Autodesk Inventor part; units mm, degrees
(part 4 of 4)
  line L177 (-517.1372, 1.22) -> (-517.8628, 1.22)
  arc A519 (-517.8628, 1.22) -> (-518.1122, 0.9525) centre (-517.8628, 0.97) ccw
  arc A520 (-519.8878, 0.9525) -> (-518.1122, 0.9525) centre (-519, 0.89) ccw
  arc A521 (-519.8878, 0.9525) -> (-520.1372, 1.22) centre (-520.1372, 0.97) ccw
  line L178 (-520.1372, 1.22) -> (-520.8628, 1.22)
  arc A522 (-520.8628, 1.22) -> (-521.1122, 0.9525) centre (-520.8628, 0.97) ccw
  arc A523 (-522.8878, 0.9525) -> (-521.1122, 0.9525) centre (-522, 0.89) ccw
  arc A524 (-522.8878, 0.9525) -> (-523.1372, 1.22) centre (-523.1372, 0.97) ccw
  line L179 (-523.1372, 1.22) -> (-523.8628, 1.22)
  arc A525 (-523.8628, 1.22) -> (-524.1122, 0.9525) centre (-523.8628, 0.97) ccw
  arc A526 (-525.8878, 0.9525) -> (-524.1122, 0.9525) centre (-525, 0.89) ccw
  arc A527 (-525.8878, 0.9525) -> (-526.1372, 1.22) centre (-526.1372, 0.97) ccw
  line L180 (-526.1372, 1.22) -> (-526.8628, 1.22)
  arc A528 (-526.8628, 1.22) -> (-527.1122, 0.9525) centre (-526.8628, 0.97) ccw
  arc A529 (-528.8878, 0.9525) -> (-527.1122, 0.9525) centre (-528, 0.89) ccw
  arc A530 (-528.8878, 0.9525) -> (-529.1372, 1.22) centre (-529.1372, 0.97) ccw
  line L181 (-529.1372, 1.22) -> (-529.8628, 1.22)
  arc A531 (-529.8628, 1.22) -> (-530.1122, 0.9525) centre (-529.8628, 0.97) ccw
  arc A532 (-531.8878, 0.9525) -> (-530.1122, 0.9525) centre (-531, 0.89) ccw
  arc A533 (-531.8878, 0.9525) -> (-532.1372, 1.22) centre (-532.1372, 0.97) ccw
  line L182 (-532.1372, 1.22) -> (-532.8628, 1.22)
  arc A534 (-532.8628, 1.22) -> (-533.1122, 0.9525) centre (-532.8628, 0.97) ccw
  arc A535 (-534.8878, 0.9525) -> (-533.1122, 0.9525) centre (-534, 0.89) ccw
  arc A536 (-534.8878, 0.9525) -> (-535.1372, 1.22) centre (-535.1372, 0.97) ccw
  line L183 (-535.1372, 1.22) -> (-535.8628, 1.22)
  arc A537 (-535.8628, 1.22) -> (-536.1122, 0.9525) centre (-535.8628, 0.97) ccw
  arc A538 (-537.8878, 0.9525) -> (-536.1122, 0.9525) centre (-537, 0.89) ccw
  arc A539 (-537.8878, 0.9525) -> (-538.1372, 1.22) centre (-538.1372, 0.97) ccw
  line L184 (-538.1372, 1.22) -> (-538.8628, 1.22)
  arc A540 (-538.8628, 1.22) -> (-539.1122, 0.9525) centre (-538.8628, 0.97) ccw
  arc A541 (-540.8878, 0.9525) -> (-539.1122, 0.9525) centre (-540, 0.89) ccw
  arc A542 (-540.8878, 0.9525) -> (-541.1372, 1.22) centre (-541.1372, 0.97) ccw
  line L185 (-541.1372, 1.22) -> (-541.8628, 1.22)
  arc A543 (-541.8628, 1.22) -> (-542.1122, 0.9525) centre (-541.8628, 0.97) ccw
  arc A544 (-543.8878, 0.9525) -> (-542.1122, 0.9525) centre (-543, 0.89) ccw
  arc A545 (-543.8878, 0.9525) -> (-544.1372, 1.22) centre (-544.1372, 0.97) ccw
  line L186 (-544.1372, 1.22) -> (-544.8628, 1.22)
  arc A546 (-544.8628, 1.22) -> (-545.1122, 0.9525) centre (-544.8628, 0.97) ccw
  arc A547 (-546.8878, 0.9525) -> (-545.1122, 0.9525) centre (-546, 0.89) ccw
  arc A548 (-546.8878, 0.9525) -> (-547.1372, 1.22) centre (-547.1372, 0.97) ccw
  line L187 (-547.1372, 1.22) -> (-547.8628, 1.22)
  arc A549 (-547.8628, 1.22) -> (-548.1122, 0.9525) centre (-547.8628, 0.97) ccw
  arc A550 (-549.8878, 0.9525) -> (-548.1122, 0.9525) centre (-549, 0.89) ccw
  arc A551 (-549.8878, 0.9525) -> (-550.1372, 1.22) centre (-550.1372, 0.97) ccw
  line L188 (-550.1372, 1.22) -> (-550.8628, 1.22)
  arc A552 (-550.8628, 1.22) -> (-551.1122, 0.9525) centre (-550.8628, 0.97) ccw
  arc A553 (-552.8878, 0.9525) -> (-551.1122, 0.9525) centre (-552, 0.89) ccw
  arc A554 (-552.8878, 0.9525) -> (-553.1372, 1.22) centre (-553.1372, 0.97) ccw
  line L189 (-553.1372, 1.22) -> (-553.8628, 1.22)
  arc A555 (-553.8628, 1.22) -> (-554.1122, 0.9525) centre (-553.8628, 0.97) ccw
  arc A556 (-555.8878, 0.9525) -> (-554.1122, 0.9525) centre (-555, 0.89) ccw
  arc A557 (-555.8878, 0.9525) -> (-556.1372, 1.22) centre (-556.1372, 0.97) ccw
  line L190 (-556.1372, 1.22) -> (-556.8628, 1.22)
  arc A558 (-556.8628, 1.22) -> (-557.1122, 0.9525) centre (-556.8628, 0.97) ccw
  arc A559 (-558.8878, 0.9525) -> (-557.1122, 0.9525) centre (-558, 0.89) ccw
  arc A560 (-558.8878, 0.9525) -> (-559.1372, 1.22) centre (-559.1372, 0.97) ccw
  line L191 (-559.1372, 1.22) -> (-559.8628, 1.22)
  arc A561 (-559.8628, 1.22) -> (-560.1122, 0.9525) centre (-559.8628, 0.97) ccw
  arc A562 (-561.8878, 0.9525) -> (-560.1122, 0.9525) centre (-561, 0.89) ccw
  arc A563 (-561.8878, 0.9525) -> (-562.1372, 1.22) centre (-562.1372, 0.97) ccw
  line L192 (-562.1372, 1.22) -> (-562.8628, 1.22)
  arc A564 (-562.8628, 1.22) -> (-563.1122, 0.9525) centre (-562.8628, 0.97) ccw
  arc A565 (-564.8878, 0.9525) -> (-563.1122, 0.9525) centre (-564, 0.89) ccw
  arc A566 (-564.8878, 0.9525) -> (-565.1372, 1.22) centre (-565.1372, 0.97) ccw
  line L193 (-565.1372, 1.22) -> (-565.8628, 1.22)
  arc A567 (-565.8628, 1.22) -> (-566.1122, 0.9525) centre (-565.8628, 0.97) ccw
  arc A568 (-567.8878, 0.9525) -> (-566.1122, 0.9525) centre (-567, 0.89) ccw
  arc A569 (-567.8878, 0.9525) -> (-568.1372, 1.22) centre (-568.1372, 0.97) ccw
  line L194 (-568.1372, 1.22) -> (-568.8628, 1.22)
  arc A570 (-568.8628, 1.22) -> (-569.1122, 0.9525) centre (-568.8628, 0.97) ccw
  arc A571 (-570.8878, 0.9525) -> (-569.1122, 0.9525) centre (-570, 0.89) ccw
  arc A572 (-570.8878, 0.9525) -> (-571.1372, 1.22) centre (-571.1372, 0.97) ccw
  line L195 (-571.1372, 1.22) -> (-571.8628, 1.22)
  arc A573 (-571.8628, 1.22) -> (-572.1122, 0.9525) centre (-571.8628, 0.97) ccw
  arc A574 (-573.8878, 0.9525) -> (-572.1122, 0.9525) centre (-573, 0.89) ccw
  arc A575 (-573.8878, 0.9525) -> (-574.1372, 1.22) centre (-574.1372, 0.97) ccw
  line L196 (-574.1372, 1.22) -> (-574.8628, 1.22)
  arc A576 (-574.8628, 1.22) -> (-575.1122, 0.9525) centre (-574.8628, 0.97) ccw
  arc A577 (-576.8878, 0.9525) -> (-575.1122, 0.9525) centre (-576, 0.89) ccw
  arc A578 (-576.8878, 0.9525) -> (-577.1372, 1.22) centre (-577.1372, 0.97) ccw
  line L197 (-577.1372, 1.22) -> (-577.8628, 1.22)
  arc A579 (-577.8628, 1.22) -> (-578.1122, 0.9525) centre (-577.8628, 0.97) ccw
  arc A580 (-579.8878, 0.9525) -> (-578.1122, 0.9525) centre (-579, 0.89) ccw
  arc A581 (-579.8878, 0.9525) -> (-580.1372, 1.22) centre (-580.1372, 0.97) ccw
  line L198 (-580.1372, 1.22) -> (-580.8628, 1.22)
  arc A582 (-580.8628, 1.22) -> (-581.1122, 0.9525) centre (-580.8628, 0.97) ccw
  arc A583 (-582.8878, 0.9525) -> (-581.1122, 0.9525) centre (-582, 0.89) ccw
  arc A584 (-582.8878, 0.9525) -> (-583.1372, 1.22) centre (-583.1372, 0.97) ccw
  line L199 (-583.1372, 1.22) -> (-583.8628, 1.22)
  arc A585 (-583.8628, 1.22) -> (-584.1122, 0.9525) centre (-583.8628, 0.97) ccw
  arc A586 (-585.8878, 0.9525) -> (-584.1122, 0.9525) centre (-585, 0.89) ccw
  arc A587 (-585.8878, 0.9525) -> (-586.1372, 1.22) centre (-586.1372, 0.97) ccw
  line L200 (-586.1372, 1.22) -> (-586.8628, 1.22)
  arc A588 (-586.8628, 1.22) -> (-587.1122, 0.9525) centre (-586.8628, 0.97) ccw
  arc A589 (-588.8878, 0.9525) -> (-587.1122, 0.9525) centre (-588, 0.89) ccw
  arc A590 (-588.8878, 0.9525) -> (-589.1372, 1.22) centre (-589.1372, 0.97) ccw
  line L201 (-589.1372, 1.22) -> (-589.8628, 1.22)
  arc A591 (-589.8628, 1.22) -> (-590.1122, 0.9525) centre (-589.8628, 0.97) ccw
  arc A592 (-591.8878, 0.9525) -> (-590.1122, 0.9525) centre (-591, 0.89) ccw
  arc A593 (-591.8878, 0.9525) -> (-592.1372, 1.22) centre (-592.1372, 0.97) ccw
  line L202 (-592.1372, 1.22) -> (-592.8628, 1.22)
  arc A594 (-592.8628, 1.22) -> (-593.1122, 0.9525) centre (-592.8628, 0.97) ccw
  arc A595 (-594.8878, 0.9525) -> (-593.1122, 0.9525) centre (-594, 0.89) ccw
  arc A596 (-594.8878, 0.9525) -> (-595.1372, 1.22) centre (-595.1372, 0.97) ccw
  line L203 (-595.1372, 1.22) -> (-595.8628, 1.22)
  arc A597 (-595.8628, 1.22) -> (-596.1122, 0.9525) centre (-595.8628, 0.97) ccw
  arc A598 (-597.8878, 0.9525) -> (-596.1122, 0.9525) centre (-597, 0.89) ccw
  arc A599 (-597.8878, 0.9525) -> (-598.1372, 1.22) centre (-598.1372, 0.97) ccw
  line L204 (-598.1372, 1.22) -> (-598.8628, 1.22)
  arc A600 (-598.8628, 1.22) -> (-599.1122, 0.9525) centre (-598.8628, 0.97) ccw
  arc A601 (-600.8878, 0.9525) -> (-599.1122, 0.9525) centre (-600, 0.89) ccw
  arc A602 (-600.8878, 0.9525) -> (-601.1372, 1.22) centre (-601.1372, 0.97) ccw
  line L205 (-601.1372, 1.22) -> (-601.8628, 1.22)
  arc A603 (-601.8628, 1.22) -> (-602.1122, 0.9525) centre (-601.8628, 0.97) ccw
  arc A604 (-603.8878, 0.9525) -> (-602.1122, 0.9525) centre (-603, 0.89) ccw
  arc A605 (-603.8878, 0.9525) -> (-604.1372, 1.22) centre (-604.1372, 0.97) ccw
  line L206 (-604.1372, 1.22) -> (-604.8628, 1.22)
  arc A606 (-604.8628, 1.22) -> (-605.1122, 0.9525) centre (-604.8628, 0.97) ccw
  arc A607 (-606.8878, 0.9525) -> (-605.1122, 0.9525) centre (-606, 0.89) ccw
  arc A608 (-606.8878, 0.9525) -> (-607.1372, 1.22) centre (-607.1372, 0.97) ccw
  line L207 (-607.1372, 1.22) -> (-607.8628, 1.22)
  arc A609 (-607.8628, 1.22) -> (-608.1122, 0.9525) centre (-607.8628, 0.97) ccw
  arc A610 (-609.8878, 0.9525) -> (-608.1122, 0.9525) centre (-609, 0.89) ccw
  arc A611 (-609.8878, 0.9525) -> (-610.1372, 1.22) centre (-610.1372, 0.97) ccw
  line L208 (-610.1372, 1.22) -> (-610.8628, 1.22)
  arc A612 (-610.8628, 1.22) -> (-611.1122, 0.9525) centre (-610.8628, 0.97) ccw
  arc A613 (-612.8878, 0.9525) -> (-611.1122, 0.9525) centre (-612, 0.89) ccw
  arc A614 (-612.8878, 0.9525) -> (-613.1372, 1.22) centre (-613.1372, 0.97) ccw
  line L209 (-613.1372, 1.22) -> (-613.8628, 1.22)
  arc A615 (-613.8628, 1.22) -> (-614.1122, 0.9525) centre (-613.8628, 0.97) ccw
  arc A616 (-615.8878, 0.9525) -> (-614.1122, 0.9525) centre (-615, 0.89) ccw
  arc A617 (-615.8878, 0.9525) -> (-616.1372, 1.22) centre (-616.1372, 0.97) ccw
  line L210 (-616.1372, 1.22) -> (-616.8628, 1.22)
  arc A618 (-616.8628, 1.22) -> (-617.1122, 0.9525) centre (-616.8628, 0.97) ccw
  arc A619 (-618.8878, 0.9525) -> (-617.1122, 0.9525) centre (-618, 0.89) ccw
  arc A620 (-618.8878, 0.9525) -> (-619.1372, 1.22) centre (-619.1372, 0.97) ccw
  line L211 (-619.1372, 1.22) -> (-619.8628, 1.22)
  arc A621 (-619.8628, 1.22) -> (-620.1122, 0.9525) centre (-619.8628, 0.97) ccw
  arc A622 (-621.8878, 0.9525) -> (-620.1122, 0.9525) centre (-621, 0.89) ccw
  arc A623 (-621.8878, 0.9525) -> (-622.1372, 1.22) centre (-622.1372, 0.97) ccw
  line L212 (-622.1372, 1.22) -> (-622.8628, 1.22)
  arc A624 (-622.8628, 1.22) -> (-623.1122, 0.9525) centre (-622.8628, 0.97) ccw
  arc A625 (-624.8878, 0.9525) -> (-623.1122, 0.9525) centre (-624, 0.89) ccw
  arc A626 (-624.8878, 0.9525) -> (-625.1372, 1.22) centre (-625.1372, 0.97) ccw
  line L213 (-625.1372, 1.22) -> (-625.8628, 1.22)
  arc A627 (-625.8628, 1.22) -> (-626.1122, 0.9525) centre (-625.8628, 0.97) ccw
  arc A628 (-627.8878, 0.9525) -> (-626.1122, 0.9525) centre (-627, 0.89) ccw
  arc A629 (-627.8878, 0.9525) -> (-628.1372, 1.22) centre (-628.1372, 0.97) ccw
  line L214 (-628.1372, 1.22) -> (-628.8628, 1.22)
  arc A630 (-628.8628, 1.22) -> (-629.1122, 0.9525) centre (-628.8628, 0.97) ccw
  arc A631 (-630.8878, 0.9525) -> (-629.1122, 0.9525) centre (-630, 0.89) ccw
  arc A632 (-630.8878, 0.9525) -> (-631.1372, 1.22) centre (-631.1372, 0.97) ccw
  line L215 (-631.1372, 1.22) -> (-631.8628, 1.22)
  arc A633 (-631.8628, 1.22) -> (-632.1122, 0.9525) centre (-631.8628, 0.97) ccw
  arc A634 (-633.8878, 0.9525) -> (-632.1122, 0.9525) centre (-633, 0.89) ccw
  arc A635 (-633.8878, 0.9525) -> (-634.1372, 1.22) centre (-634.1372, 0.97) ccw
  line L216 (-634.1372, 1.22) -> (-634.8628, 1.22)
  arc A636 (-634.8628, 1.22) -> (-635.1122, 0.9525) centre (-634.8628, 0.97) ccw
  arc A637 (-636.8878, 0.9525) -> (-635.1122, 0.9525) centre (-636, 0.89) ccw
  arc A638 (-636.8878, 0.9525) -> (-637.1372, 1.22) centre (-637.1372, 0.97) ccw
  line L217 (-637.1372, 1.22) -> (-637.8628, 1.22)
  arc A639 (-637.8628, 1.22) -> (-638.1122, 0.9525) centre (-637.8628, 0.97) ccw
  arc A640 (-639.8878, 0.9525) -> (-638.1122, 0.9525) centre (-639, 0.89) ccw
  arc A641 (-639.8878, 0.9525) -> (-640.1372, 1.22) centre (-640.1372, 0.97) ccw
  line L218 (-640.1372, 1.22) -> (-640.8628, 1.22)
  arc A642 (-640.8628, 1.22) -> (-641.1122, 0.9525) centre (-640.8628, 0.97) ccw
  arc A643 (-642.8878, 0.9525) -> (-641.1122, 0.9525) centre (-642, 0.89) ccw
  arc A644 (-642.8878, 0.9525) -> (-643.1372, 1.22) centre (-643.1372, 0.97) ccw
  line L219 (-643.1372, 1.22) -> (-643.8628, 1.22)
  arc A645 (-643.8628, 1.22) -> (-644.1122, 0.9525) centre (-643.8628, 0.97) ccw
  arc A646 (-645.8878, 0.9525) -> (-644.1122, 0.9525) centre (-645, 0.89) ccw
  arc A647 (-645.8878, 0.9525) -> (-646.1372, 1.22) centre (-646.1372, 0.97) ccw
  line L220 (-646.1372, 1.22) -> (-646.8628, 1.22)
  arc A648 (-646.8628, 1.22) -> (-647.1122, 0.9525) centre (-646.8628, 0.97) ccw
  arc A649 (-648.8878, 0.9525) -> (-647.1122, 0.9525) centre (-648, 0.89) ccw
  arc A650 (-648.8878, 0.9525) -> (-649.1372, 1.22) centre (-649.1372, 0.97) ccw
  line L221 (-649.1372, 1.22) -> (-649.8628, 1.22)
  arc A651 (-649.8628, 1.22) -> (-650.1122, 0.9525) centre (-649.8628, 0.97) ccw
  arc A652 (-651.8878, 0.9525) -> (-650.1122, 0.9525) centre (-651, 0.89) ccw
  arc A653 (-651.8878, 0.9525) -> (-652.1372, 1.22) centre (-652.1372, 0.97) ccw
  line L222 (-652.1372, 1.22) -> (-652.8628, 1.22)
  arc A654 (-652.8628, 1.22) -> (-653.1122, 0.9525) centre (-652.8628, 0.97) ccw
  arc A655 (-654.8878, 0.9525) -> (-653.1122, 0.9525) centre (-654, 0.89) ccw
  arc A656 (-654.8878, 0.9525) -> (-655.1372, 1.22) centre (-655.1372, 0.97) ccw
  line L223 (-655.1372, 1.22) -> (-655.8628, 1.22)
  arc A657 (-655.8628, 1.22) -> (-656.1122, 0.9525) centre (-655.8628, 0.97) ccw
  arc A658 (-657.8878, 0.9525) -> (-656.1122, 0.9525) centre (-657, 0.89) ccw
  arc A659 (-657.8878, 0.9525) -> (-658.1372, 1.22) centre (-658.1372, 0.97) ccw
  line L224 (-658.1372, 1.22) -> (-658.8628, 1.22)
  arc A660 (-658.8628, 1.22) -> (-659.1122, 0.9525) centre (-658.8628, 0.97) ccw
  arc A661 (-660.8878, 0.9525) -> (-659.1122, 0.9525) centre (-660, 0.89) ccw
  arc A662 (-660.8878, 0.9525) -> (-661.1372, 1.22) centre (-661.1372, 0.97) ccw
  line L225 (-661.1372, 1.22) -> (-661.8628, 1.22)
  arc A663 (-661.8628, 1.22) -> (-662.1122, 0.9525) centre (-661.8628, 0.97) ccw
  arc A664 (-663.8878, 0.9525) -> (-662.1122, 0.9525) centre (-663, 0.89) ccw
  arc A665 (-663.8878, 0.9525) -> (-664.1372, 1.22) centre (-664.1372, 0.97) ccw
  line L226 (-664.1372, 1.22) -> (-664.8628, 1.22)
  arc A666 (-664.8628, 1.22) -> (-665.1122, 0.9525) centre (-664.8628, 0.97) ccw
  arc A667 (-666.8878, 0.9525) -> (-665.1122, 0.9525) centre (-666, 0.89) ccw
  arc A668 (-666.8878, 0.9525) -> (-667.1372, 1.22) centre (-667.1372, 0.97) ccw
  line L227 (-667.1372, 1.22) -> (-667.8628, 1.22)
  arc A669 (-667.8628, 1.22) -> (-668.1122, 0.9525) centre (-667.8628, 0.97) ccw
  arc A670 (-669.8878, 0.9525) -> (-668.1122, 0.9525) centre (-669, 0.89) ccw
  arc A671 (-669.8878, 0.9525) -> (-670.1372, 1.22) centre (-670.1372, 0.97) ccw
  line L228 (-670.1372, 1.22) -> (-670.8628, 1.22)
  arc A672 (-670.8628, 1.22) -> (-671.1122, 0.9525) centre (-670.8628, 0.97) ccw
  arc A673 (-672.8878, 0.9525) -> (-671.1122, 0.9525) centre (-672, 0.89) ccw
  arc A674 (-672.8878, 0.9525) -> (-673.1372, 1.22) centre (-673.1372, 0.97) ccw
  line L229 (-673.1372, 1.22) -> (-673.8628, 1.22)
  arc A675 (-673.8628, 1.22) -> (-674.1122, 0.9525) centre (-673.8628, 0.97) ccw
  arc A676 (-675.8878, 0.9525) -> (-674.1122, 0.9525) centre (-675, 0.89) ccw
  arc A677 (-675.8878, 0.9525) -> (-676.1372, 1.22) centre (-676.1372, 0.97) ccw
  line L230 (-676.1372, 1.22) -> (-676.8628, 1.22)
  arc A678 (-676.8628, 1.22) -> (-677.1122, 0.9525) centre (-676.8628, 0.97) ccw
  arc A679 (-678.8878, 0.9525) -> (-677.1122, 0.9525) centre (-678, 0.89) ccw
  arc A680 (-678.8878, 0.9525) -> (-679.1372, 1.22) centre (-679.1372, 0.97) ccw
  line L231 (-679.1372, 1.22) -> (-679.8628, 1.22)
  arc A681 (-679.8628, 1.22) -> (-680.1122, 0.9525) centre (-679.8628, 0.97) ccw
  arc A682 (-681.8878, 0.9525) -> (-680.1122, 0.9525) centre (-681, 0.89) ccw
  arc A683 (-681.8878, 0.9525) -> (-682.1372, 1.22) centre (-682.1372, 0.97) ccw
  line L232 (-682.1372, 1.22) -> (-682.8628, 1.22)
  arc A684 (-682.8628, 1.22) -> (-683.1122, 0.9525) centre (-682.8628, 0.97) ccw
  arc A685 (-684.8878, 0.9525) -> (-683.1122, 0.9525) centre (-684, 0.89) ccw
  arc A686 (-684.8878, 0.9525) -> (-685.1372, 1.22) centre (-685.1372, 0.97) ccw
  line L233 (-685.1372, 1.22) -> (-685.8628, 1.22)
  arc A687 (-685.8628, 1.22) -> (-686.1122, 0.9525) centre (-685.8628, 0.97) ccw
  arc A688 (-687.8878, 0.9525) -> (-686.1122, 0.9525) centre (-687, 0.89) ccw
  arc A689 (-687.8878, 0.9525) -> (-688.1372, 1.22) centre (-688.1372, 0.97) ccw
  line L234 (-688.1372, 1.22) -> (-688.8628, 1.22)
  arc A690 (-688.8628, 1.22) -> (-689.1122, 0.9525) centre (-688.8628, 0.97) ccw
  arc A691 (-690.8878, 0.9525) -> (-689.1122, 0.9525) centre (-690, 0.89) ccw
  arc A692 (-690.8878, 0.9525) -> (-691.1372, 1.22) centre (-691.1372, 0.97) ccw
  line L235 (-691.1372, 1.22) -> (-691.8628, 1.22)
  arc A693 (-691.8628, 1.22) -> (-692.1122, 0.9525) centre (-691.8628, 0.97) ccw
  arc A694 (-693.8878, 0.9525) -> (-692.1122, 0.9525) centre (-693, 0.89) ccw
  arc A695 (-693.8878, 0.9525) -> (-694.1372, 1.22) centre (-694.1372, 0.97) ccw
  line L236 (-694.1372, 1.22) -> (-694.8628, 1.22)
  arc A696 (-694.8628, 1.22) -> (-695.1122, 0.9525) centre (-694.8628, 0.97) ccw
  arc A697 (-696.8878, 0.9525) -> (-695.1122, 0.9525) centre (-696, 0.89) ccw
  arc A698 (-696.8878, 0.9525) -> (-697.1372, 1.22) centre (-697.1372, 0.97) ccw
  line L237 (-697.1372, 1.22) -> (-697.8628, 1.22)
  arc A699 (-697.8628, 1.22) -> (-698.1122, 0.9525) centre (-697.8628, 0.97) ccw
  arc A700 (-699.8878, 0.9525) -> (-698.1122, 0.9525) centre (-699, 0.89) ccw
  arc A701 (-699.8878, 0.9525) -> (-700.1372, 1.22) centre (-700.1372, 0.97) ccw
  line L238 (-700.1372, 1.22) -> (-700.8628, 1.22)
  arc A702 (-700.8628, 1.22) -> (-701.1122, 0.9525) centre (-700.8628, 0.97) ccw
  arc A703 (-702.8878, 0.9525) -> (-701.1122, 0.9525) centre (-702, 0.89) ccw
  arc A704 (-702.8878, 0.9525) -> (-703.1372, 1.22) centre (-703.1372, 0.97) ccw
  line L239 (-703.1372, 1.22) -> (-703.8628, 1.22)
  arc A705 (-703.8628, 1.22) -> (-704.1122, 0.9525) centre (-703.8628, 0.97) ccw
  arc A706 (-705.8878, 0.9525) -> (-704.1122, 0.9525) centre (-705, 0.89) ccw
  arc A707 (-705.8878, 0.9525) -> (-706.1372, 1.22) centre (-706.1372, 0.97) ccw
  line L240 (-706.1372, 1.22) -> (-706.8628, 1.22)
  arc A708 (-706.8628, 1.22) -> (-707.1122, 0.9525) centre (-706.8628, 0.97) ccw
  arc A709 (-708.8878, 0.9525) -> (-707.1122, 0.9525) centre (-708, 0.89) ccw
  arc A710 (-708.8878, 0.9525) -> (-709.1372, 1.22) centre (-709.1372, 0.97) ccw
  line L241 (-709.1372, 1.22) -> (-709.8628, 1.22)
  arc A711 (-709.8628, 1.22) -> (-710.1122, 0.9525) centre (-709.8628, 0.97) ccw
  arc A712 (-711.8878, 0.9525) -> (-710.1122, 0.9525) centre (-711, 0.89) ccw
  arc A713 (-711.8878, 0.9525) -> (-712.1372, 1.22) centre (-712.1372, 0.97) ccw
  line L242 (-712.1372, 1.22) -> (-712.8628, 1.22)
  arc A714 (-712.8628, 1.22) -> (-713.1122, 0.9525) centre (-712.8628, 0.97) ccw
  arc A715 (-714.8878, 0.9525) -> (-713.1122, 0.9525) centre (-714, 0.89) ccw
  arc A716 (-714.8878, 0.9525) -> (-715.1372, 1.22) centre (-715.1372, 0.97) ccw
  line L243 (-715.1372, 1.22) -> (-715.8628, 1.22)
  arc A717 (-715.8628, 1.22) -> (-716.1122, 0.9525) centre (-715.8628, 0.97) ccw
  arc A718 (-717.8878, 0.9525) -> (-716.1122, 0.9525) centre (-717, 0.89) ccw
  arc A719 (-717.8878, 0.9525) -> (-718.1372, 1.22) centre (-718.1372, 0.97) ccw
  line L244 (-718.1372, 1.22) -> (-718.8628, 1.22)
  arc A720 (-718.8628, 1.22) -> (-719.1122, 0.9525) centre (-718.8628, 0.97) ccw
  arc A721 (-720.8878, 0.9525) -> (-719.1122, 0.9525) centre (-720, 0.89) ccw
  arc A722 (-720.8878, 0.9525) -> (-721.1372, 1.22) centre (-721.1372, 0.97) ccw
  line L245 (-721.1372, 1.22) -> (-721.8628, 1.22)
  arc A723 (-721.8628, 1.22) -> (-722.1122, 0.9525) centre (-721.8628, 0.97) ccw
  arc A724 (-723.8878, 0.9525) -> (-722.1122, 0.9525) centre (-723, 0.89) ccw
  arc A725 (-723.8878, 0.9525) -> (-724.1372, 1.22) centre (-724.1372, 0.97) ccw
  line L246 (-724.1372, 1.22) -> (-724.8628, 1.22)
  arc A726 (-724.8628, 1.22) -> (-725.1122, 0.9525) centre (-724.8628, 0.97) ccw
  arc A727 (-726.8878, 0.9525) -> (-725.1122, 0.9525) centre (-726, 0.89) ccw
  arc A728 (-726.8878, 0.9525) -> (-727.1372, 1.22) centre (-727.1372, 0.97) ccw
  line L247 (-727.1372, 1.22) -> (-727.8628, 1.22)
  arc A729 (-727.8628, 1.22) -> (-728.1122, 0.9525) centre (-727.8628, 0.97) ccw
  arc A730 (-729.8878, 0.9525) -> (-728.1122, 0.9525) centre (-729, 0.89) ccw
  arc A731 (-729.8878, 0.9525) -> (-730.1372, 1.22) centre (-730.1372, 0.97) ccw
  line L248 (-730.1372, 1.22) -> (-730.8628, 1.22)
  arc A732 (-730.8628, 1.22) -> (-731.1122, 0.9525) centre (-730.8628, 0.97) ccw
  arc A733 (-732.8878, 0.9525) -> (-731.1122, 0.9525) centre (-732, 0.89) ccw
  arc A734 (-732.8878, 0.9525) -> (-733.1372, 1.22) centre (-733.1372, 0.97) ccw
  line L249 (-733.1372, 1.22) -> (-733.8628, 1.22)
  arc A735 (-733.8628, 1.22) -> (-734.1122, 0.9525) centre (-733.8628, 0.97) ccw
  arc A736 (-735.8878, 0.9525) -> (-734.1122, 0.9525) centre (-735, 0.89) ccw
  arc A737 (-735.8878, 0.9525) -> (-736.1372, 1.22) centre (-736.1372, 0.97) ccw
  line L250 (-736.1372, 1.22) -> (-736.8628, 1.22)
  arc A738 (-736.8628, 1.22) -> (-737.1122, 0.9525) centre (-736.8628, 0.97) ccw
  arc A739 (-738.8878, 0.9525) -> (-737.1122, 0.9525) centre (-738, 0.89) ccw
  arc A740 (-738.8878, 0.9525) -> (-739.1372, 1.22) centre (-739.1372, 0.97) ccw
  line L251 (-739.1372, 1.22) -> (-739.8628, 1.22)
  arc A741 (-739.8628, 1.22) -> (-740.1122, 0.9525) centre (-739.8628, 0.97) ccw
  arc A742 (-741.8878, 0.9525) -> (-740.1122, 0.9525) centre (-741, 0.89) ccw
  arc A743 (-741.8878, 0.9525) -> (-742.1372, 1.22) centre (-742.1372, 0.97) ccw
  line L252 (-742.1372, 1.22) -> (-742.8628, 1.22)
  arc A744 (-742.8628, 1.22) -> (-743.1122, 0.9525) centre (-742.8628, 0.97) ccw
  arc A745 (-744.8878, 0.9525) -> (-743.1122, 0.9525) centre (-744, 0.89) ccw
  arc A746 (-744.8878, 0.9525) -> (-745.1372, 1.22) centre (-745.1372, 0.97) ccw
  line L253 (-745.1372, 1.22) -> (-745.8628, 1.22)
  arc A747 (-745.8628, 1.22) -> (-746.1122, 0.9525) centre (-745.8628, 0.97) ccw
  arc A748 (-747.8878, 0.9525) -> (-746.1122, 0.9525) centre (-747, 0.89) ccw
  arc A749 (-747.8878, 0.9525) -> (-748.1372, 1.22) centre (-748.1372, 0.97) ccw
  line L254 (-748.1372, 1.22) -> (-748.8628, 1.22)
  arc A750 (-748.8628, 1.22) -> (-749.1122, 0.9525) centre (-748.8628, 0.97) ccw
  arc A751 (-750.8878, 0.9525) -> (-749.1122, 0.9525) centre (-750, 0.89) ccw
  arc A752 (-750.8878, 0.9525) -> (-751.1372, 1.22) centre (-751.1372, 0.97) ccw
  line L255 (-751.1372, 1.22) -> (-751.8628, 1.22)
  arc A753 (-751.8628, 1.22) -> (-752.1122, 0.9525) centre (-751.8628, 0.97) ccw
  arc A754 (-753.8878, 0.9525) -> (-752.1122, 0.9525) centre (-753, 0.89) ccw
  arc A755 (-753.8878, 0.9525) -> (-754.1372, 1.22) centre (-754.1372, 0.97) ccw
  line L256 (-754.1372, 1.22) -> (-754.8628, 1.22)
  arc A756 (-754.8628, 1.22) -> (-755.1122, 0.9525) centre (-754.8628, 0.97) ccw
  arc A757 (-756.8878, 0.9525) -> (-755.1122, 0.9525) centre (-756, 0.89) ccw
  arc A758 (-756.8878, 0.9525) -> (-757.1372, 1.22) centre (-757.1372, 0.97) ccw
  line L257 (-757.1372, 1.22) -> (-757.8628, 1.22)
  arc A759 (-757.8628, 1.22) -> (-758.1122, 0.9525) centre (-757.8628, 0.97) ccw
  arc A760 (-759.8878, 0.9525) -> (-758.1122, 0.9525) centre (-759, 0.89) ccw
  arc A761 (-759.8878, 0.9525) -> (-760.1372, 1.22) centre (-760.1372, 0.97) ccw
  line L258 (-760.1372, 1.22) -> (-760.8628, 1.22)
  arc A762 (-760.8628, 1.22) -> (-761.1122, 0.9525) centre (-760.8628, 0.97) ccw
  arc A763 (-762.8878, 0.9525) -> (-761.1122, 0.9525) centre (-762, 0.89) ccw
  arc A764 (-762.8878, 0.9525) -> (-763.1372, 1.22) centre (-763.1372, 0.97) ccw
  line L259 (-763.1372, 1.22) -> (-763.8628, 1.22)
  arc A765 (-763.8628, 1.22) -> (-764.1122, 0.9525) centre (-763.8628, 0.97) ccw
  arc A766 (-765.8878, 0.9525) -> (-764.1122, 0.9525) centre (-765, 0.89) ccw
  arc A767 (-765.8878, 0.9525) -> (-766.1372, 1.22) centre (-766.1372, 0.97) ccw
  line L260 (-766.1372, 1.22) -> (-766.8628, 1.22)
  arc A768 (-766.8628, 1.22) -> (-767.1122, 0.9525) centre (-766.8628, 0.97) ccw
  arc A769 (-768, 0) -> (-767.1122, 0.9525) centre (-768, 0.89) ccw
  point P0 (0, 0)
  constraints: 899 symmetric about line, 770 point on circle, 385 centre point, 260 end point, 385 other
extrude "Extrusion3" add sketch "Sketch3" against normal blind 15 contours L2 A385 A386 L133 A387 A388 A389 L134 A390 A391 A392 L135 A393 A394 A395 L136 A396 A397 A398 L137 A399 A400 A401 L138 A402 A403 A404 L139 A405 A406 A407 L140 A408 A409 A410 L141 A411 A412 A413 L142 A414 A415 A416 L143 A417 A418 A419 L144 A420 A421 A422 L145 A423 A424 A425 L146 A426 A427 A428 L147 A429 A430 A431 L148 A432 A433 A434 L149 A435 A436 A437 L150 A438 A439 A440 L151 A441 A442 A443 L152 A444 A445 A446 L153 A447 A448 A449 L154 A450 A451 A452 L155 A453 A454 A455 L156 A456 A457 A458 L157 A459 A460 A461 L158 A462 A463 A464 L159 A465 A466 A467 L160 A468 A469 A470 L161 A471 A472 A473 L162 A474 A475 A476 L163 A477 A478 A479 L164 A480 A481 A482 L165 A483 A484 A485 L166 A486 A487 A488 L167 A489 A490 A491 L168 A492 A493 A494 L169 A495 A496 A497 L170 A498 A499 A500 L171 A501 A502 A503 L172 A504 A505 A506 L173 A507 A508 A509 L174 A510 A511 A512 L175 A513 A514 A515 L176 A516 A517 A518 L177 A519 A520 A521 L178 A522 A523 A524 L179 A525 A526 A527 L180 A528 A529 A530 L181 A531 A532 A533 L182 A534 A535 A536 L183 A537 A538 A539 L184 A540 A541 A542 L185 A543 A544 A545 L186 A546 A547 A548 L187 A549 A550 A551 L188 A552 A553 A554 L189 A555 A556 A557 L190 A558 A559 A560 L191 A561 A562 A563 L192 A564 A565 A566 L193 A567 A568 A569 L194 A570 A571 A572 L195 A573 A574 A575 L196 A576 A577 A578 L197 A579 A580 A581 L198 A582 A583 A584 L199 A585 A586 A587 L200 A588 A589 A590 L201 A591 A592 A593 L202 A594 A595 A596 L203 A597 A598 A599 L204 A600 A601 A602 L205 A603 A604 A605 L206 A606 A607 A608 L207 A609 A610 A611 L208 A612 A613 A614 L209 A615 A616 A617 L210 A618 A619 A620 L211 A621 A622 A623 L212 A624 A625 A626 L213 A627 A628 A629 L214 A630 A631 A632 L215 A633 A634 A635 L216 A636 A637 A638 L217 A639 A640 A641 L218 A642 A643 A644 L219 A645 A646 A647 L220 A648 A649 A650 L221 A651 A652 A653 L222 A654 A655 A656 L223 A657 A658 A659 L224 A660 A661 A662 L225 A663 A664 A665 L226 A666 A667 A668 L227 A669 A670 A671 L228 A672 A673 A674 L229 A675 A676 A677 L230 A678 A679 A680 L231 A681 A682 A683 L232 A684 A685 A686 L233 A687 A688 A689 L234 A690 A691 A692 L235 A693 A694 A695 L236 A696 A697 A698 L237 A699 A700 A701 L238 A702 A703 A704 L239 A705 A706 A707 L240 A708 A709 A710 L241 A711 A712 A713 L242 A714 A715 A716 L243 A717 A718 A719 L244 A720 A721 A722 L245 A723 A724 A725 L246 A726 A727 A728 L247 A729 A730 A731 L248 A732 A733 A734 L249 A735 A736 A737 L250 A738 A739 A740 L251 A741 A742 A743 L252 A744 A745 A746 L253 A747 A748 A749 L254 A750 A751 A752 L255 A753 A754 A755 L256 A756 A757 A758 L257 A759 A760 A761 L258 A762 A763 A764 L259 A765 A766 A767 L260 A768 A769 L131 L132
sketch "Sketch7" plane through (0, 0, 15) normal (0, 0, 1) x (1, 0, 0)
  line L0 (0, 2.4) -> (-3, 2.4)
  line L1 (0, 0) -> (-3, 0) construction
  line L2 (0, 2.4) -> (0, 0)
  line L3 (-3, 0) -> (-3, 2.4) construction
  arc A0 (-0.8878, 0.9525) -> (0, 0) centre (0, 0.89) ccw
  arc A1 (-3, 0) -> (-2.1122, 0.9525) centre (-3, 0.89) ccw
  line L4 (-1.1372, 1.22) -> (-1.8628, 1.22) construction
  line L5 (-1.5, 1.22) -> (-1.5, 0) construction
  line L6 (-1.8628, 1.22) -> (-1.1372, 1.22)
  arc A2 (-1.8628, 1.22) -> (-2.1122, 0.9525) centre (-1.8628, 0.97) ccw
  arc A3 (-0.8878, 0.9525) -> (-1.1372, 1.22) centre (-1.1372, 0.97) ccw
  line L7 (-6, 0) -> (-3, 0) construction
  line L8 (-4.8628, 1.22) -> (-4.1372, 1.22) construction
  line L9 (-4.5, 1.22) -> (-4.5, 0) construction
  line L10 (0, 2.4) -> (-768, 2.4) construction
  line L11 (-3, 2.4) -> (-768, 2.4) construction
  line L12 (-385.5, 2.4) -> (-385.5, -173.6917) construction
  line L13 (-771, 2.4) -> (-768, 2.4)
  line L14 (-771, 0) -> (-768, 0) construction
  line L15 (-771, 2.4) -> (-771, 0) construction
  line L16 (-768, 0) -> (-768, 2.4)
  arc A4 (-771, 0) -> (-770.1122, 0.9525) centre (-771, 0.89) ccw
  arc A5 (-768.8878, 0.9525) -> (-768, 0) centre (-768, 0.89) ccw
  line L17 (-769.8628, 1.22) -> (-769.1372, 1.22) construction
  line L18 (-769.5, 1.22) -> (-769.5, 0) construction
  line L19 (-769.1372, 1.22) -> (-769.8628, 1.22)
  arc A6 (-768.8878, 0.9525) -> (-769.1372, 1.22) centre (-769.1372, 0.97) ccw
  arc A7 (-769.8628, 1.22) -> (-770.1122, 0.9525) centre (-769.8628, 0.97) ccw
  line L20 (-765, 0) -> (-768, 0) construction
  line L21 (-766.1372, 1.22) -> (-766.8628, 1.22) construction
  line L22 (-766.5, 1.22) -> (-766.5, 0) construction
  arc A8 (-771.8878, 0.9525) -> (-771, 0) centre (-771, 0.89) ccw
  arc A9 (-771.8878, 0.9525) -> (-772.1372, 1.22) centre (-772.1372, 0.97) ccw
  line L23 (-772.5, 1.22) -> (-772.5, 0) construction
  line L24 (-771, 0) -> (-771, 2.4) construction
  line L25 (-772.8628, 1.22) -> (-772.1372, 1.22) construction
  line L26 (-772.1372, 1.22) -> (-772.8628, 1.22)
  arc A10 (-772.8628, 1.22) -> (-773.1122, 0.9525) centre (-772.8628, 0.97) ccw
  line L27 (-774, 2.4) -> (-771, 2.4)
  line L28 (-774, 2.4) -> (-774, 0) construction
  arc A11 (-774, 0) -> (-773.1122, 0.9525) centre (-774, 0.89) ccw
  line L29 (-774, 0) -> (-771, 0) construction
  arc A12 (-774.8878, 0.9525) -> (-774, 0) centre (-774, 0.89) ccw
  arc A13 (-774.8878, 0.9525) -> (-775.1372, 1.22) centre (-775.1372, 0.97) ccw
  line L30 (-775.5, 1.22) -> (-775.5, 0) construction
  line L31 (-774, 0) -> (-774, 2.4) construction
  line L32 (-775.8628, 1.22) -> (-775.1372, 1.22) construction
  line L33 (-775.1372, 1.22) -> (-775.8628, 1.22)
  arc A14 (-775.8628, 1.22) -> (-776.1122, 0.9525) centre (-775.8628, 0.97) ccw
  line L34 (-777, 2.4) -> (-774, 2.4)
  line L35 (-777, 2.4) -> (-777, 0) construction
  arc A15 (-777, 0) -> (-776.1122, 0.9525) centre (-777, 0.89) ccw
  line L36 (-777, 0) -> (-774, 0) construction
  arc A16 (-777.8878, 0.9525) -> (-777, 0) centre (-777, 0.89) ccw
  arc A17 (-777.8878, 0.9525) -> (-778.1372, 1.22) centre (-778.1372, 0.97) ccw
  line L37 (-778.5, 1.22) -> (-778.5, 0) construction
  line L38 (-777, 0) -> (-777, 2.4) construction
  line L39 (-778.8628, 1.22) -> (-778.1372, 1.22) construction
  line L40 (-778.1372, 1.22) -> (-778.8628, 1.22)
  arc A18 (-778.8628, 1.22) -> (-779.1122, 0.9525) centre (-778.8628, 0.97) ccw
  line L41 (-780, 2.4) -> (-777, 2.4)
  line L42 (-780, 2.4) -> (-780, 0)
  arc A19 (-780, 0) -> (-779.1122, 0.9525) centre (-780, 0.89) ccw
  line L43 (-780, 0) -> (-777, 0) construction
  point P0 (-777, 0)
  point P1 (-774, 0)
  dimension "d20" = 3
  dimension "d21" = 2.4
  dimension "d22" = 1.78
  dimension "d23" = 1.78
  dimension "d24" = 1.22
  dimension "d25" = 0.25
  dimension "d28" = 3
  constraints: 86 end point, 40 point on circle, 25 symmetric about line, 20 centre point, 15 point on line, 5 tangent, 3 horizontal, 3 midpoint, 2 collinear, 2 perpendicular, 1 equal radius, 1 parallel, 1 vertical, 84 other
  measures "d20" distance of L0.start L0.end
  measures "d21" distance of L1.start L0.start
  measures "d22" diameter of A0
  measures "d23" diameter of A1
  measures "d24" distance from line of L1.start L4
  measures "d25" radius of A2
  measures "d28" distance of A5.centre A8.centre
extrude "Extrusion7" add sketch "Sketch7" against normal blind 15
equation "\"d4\" = d2"
body "Solid1"
